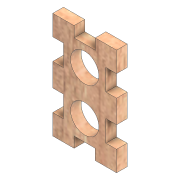
# Autodesk Inventor part: voorkant knoppendoosje
Saved by Autodesk Inventor 2020.3 (Build 243373000, 373)
## iProperties
Created: 2020-12-08
Part Number: voorkant knoppendoosje
Material: Wood (Birch)
Document SubType Name: Sheet Metal
Designer: Svend
Density: 0.55 g/cm^3
Sheet Metal Rule: Default_mm
Appearance: Birch - Natural Polished
Author: Svend
Autodesk Inventor part; units mm, degrees
ref_plane "YZ Plane" through (0, 0, 0) normal (1, 0, 0) x (0, 1, 0)
ref_plane "XZ Plane" through (0, 0, 0) normal (0, 1, 0) x (-1, 0, 0)
ref_plane "XY Plane" through (0, 0, 0) normal (0, 0, 1) x (1, 0, 0)
sketch "Sketch1" plane through (0, 0, 0) normal (0, 0, 1) x (1, 0, 0)
  circle A0 centre (0, 0) radius 8
  circle A1 centre (0, -25) radius 8
  line L0 (0, 0) -> (0, -25) construction
  line L1 (-18, 17.5) -> (18, 17.5)
  line L2 (18, 17.5) -> (18, -42.5)
  line L3 (18, -42.5) -> (-18, -42.5)
  line L4 (-18, -42.5) -> (-18, 17.5)
  line L5 (-18, 17.5) -> (18, -42.5) construction
  line L6 (18, 17.5) -> (-18, -42.5) construction
  line L7 (-6, 17.5) -> (6, 17.5)
  line L8 (6, 17.5) -> (6, 11.5)
  line L9 (6, 11.5) -> (-6, 11.5)
  line L10 (-6, 11.5) -> (-6, 17.5)
  line L11 (-6, -42.5) -> (6, -42.5)
  line L12 (6, -42.5) -> (6, -36.5)
  line L13 (6, -36.5) -> (-6, -36.5)
  line L14 (-6, -36.5) -> (-6, -42.5)
  line L15 (-18, -31) -> (-12, -31)
  line L16 (-12, -31) -> (-12, -19)
  line L17 (-12, -19) -> (-18, -19)
  line L18 (-18, -19) -> (-18, -31)
  line L19 (-18, -6) -> (-12, -6)
  line L20 (-12, -6) -> (-12, 6)
  line L21 (-12, 6) -> (-18, 6)
  line L22 (-18, 6) -> (-18, -6)
  line L23 (18, -6) -> (12, -6)
  line L24 (12, -6) -> (12, 6)
  line L25 (12, 6) -> (18, 6)
  line L26 (18, 6) -> (18, -6)
  line L27 (18, -31) -> (12, -31)
  line L28 (12, -31) -> (12, -19)
  line L29 (12, -19) -> (18, -19)
  line L30 (18, -19) -> (18, -31)
  point P0 (0, -12.5)
  point P1 (0, 11.5)
  point P2 (0, 17.5)
  point P3 (12, 0)
  point P4 (-12, 0)
  point P5 (-12, -25)
  point P6 (12, -25)
  dimension "d0" = 16
  dimension "d1" = 25
  dimension "d2" = 36
  dimension "d3" = 60
  dimension "d4" = 12
  dimension "d5" = 6
  measures "d0" diameter of A0
  measures "d1" distance of L0.end L0.start
  measures "d2" distance of L2.end L3.end
  measures "d3" distance of L1.end L2.end
  measures "d4" distance of L8.end L9.end
  measures "d5" distance of L7.end L8.end
extrude "Plate1" add sketch "Sketch1" along normal blind 6 contours L1 L10 L9 L8 L2 L25 L24 L23 L29 L28 L27 L3 L12 L13 L14 L4 L15 L16 L17 L19 L20 L21
equation "\"d7\" = Thickness"
equation "\"BendRadius\" = Thickness"
equation "\"BendReliefWidth\" = Thickness"
equation "\"BendReliefDepth\" = 0.5 * Thickness"
equation "\"CornerReliefSize\" = 4 * Thickness"
equation "\"MinimumRemnant\" = 2 * Thickness"
equation "\"TransitionRadius\" = BendRadius"
equation "\"JacobiRadiusSize\" = BendRadius"
equation "\"GapSize\" = Thickness"
equation "\"Thickness\" = 6"
body "Solid1"
